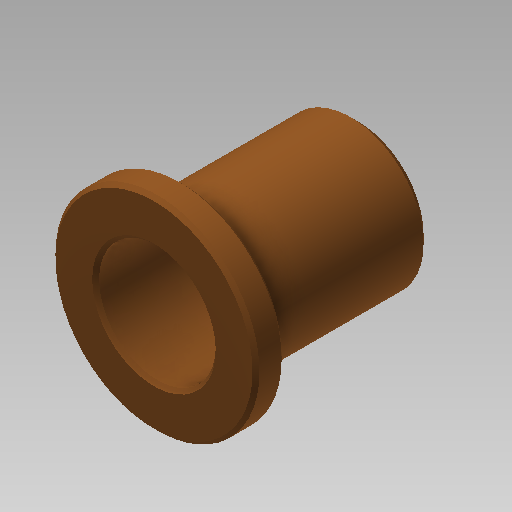
# Autodesk Inventor part: PWTR-0026
Saved by Autodesk Inventor 2020 (Build 240168000, 168)
## iProperties
Part Number: PWTR-0026
Document SubType Name: Modeling
Created: 2003-12-08
Designer: Bill Bogan
Material: Bronze, Soft Tin
Manufacturer: Standard
Standards Organization: Custom
Description: BUSHING - 1/2 ID
Density: 8.874 g/cm^3
Mass: 19.131 g
Surface Area: 25.0806 cm^2
Volume: 2.15584 cm^3
Appearance: Bronze - Satin
Vendor: Non-Design Specific
Control State: 0
Master: False
Checked Out: False
Shininess: 64.0
Length Units: 11272
Angle Units: 11279
Time Units: 11290
Mass Units: 11286
Length Display Precision: 3
Angle Display Precision: 2
Compacted: True
Today: Wednesday
Density: 0.0
Volumn: 0.0
Area: 0.0
PropertySet Name: Model Information
Author: Bill Bogan
Revision Number: B
Autodesk Inventor part; units mm, degrees
ref_plane "YZ Plane" through (0, 0, 0) normal (1, 0, 0) x (0, 1, 0)
ref_plane "XZ Plane" through (0, 0, 0) normal (0, 1, 0) x (-1, 0, 0)
ref_plane "XY Plane" through (0, 0, 0) normal (0, 0, 1) x (1, 0, 0)
sketch "Sketch1" plane through (0, 0, 0) normal (0, 0, 1) x (1, 0, 0)
  circle A0 centre (0, 0) radius 7.9375
  dimension "d0" = 15.875
  constraints: 1 centre point
  measures "d0" diameter of A0
extrude "Extrusion1" add sketch "Sketch1" along normal blind 19.05
sketch "Sketch2" plane through (0, 0, 19.05) normal (0, 0, 1) x (1, 0, 0)
  circle A0 centre (0, 0) radius 7.9375 projected
  circle A1 centre (0, 0) radius 11.1125
  dimension "d3" = 3.175
  constraints: 1 centre point
  measures "d3" radial gap between concentric circles of A0 A1
extrude "Extrusion2" add sketch "Sketch2" along normal blind 3.175 contours A0 | A1
chamfer "Chamfer1" distance 0.7937 angle 45 1 edges at (-7.9375, 0, 0)
sketch "Sketch3" plane through (0, 0, 22.225) normal (0, 0, 1) x (1, 0, 0)
  circle A0 centre (0, 0) radius 11.1125 projected
hole "Hole1" at (0, 0, 22.225) direction (0, 0, -1) diameter 12.7 end through all
chamfer "Chamfer2" distance 0.381 angle 45 2 edges at (0, 6.35, 22.225) (0, 6.35, 0)
chamfer "Chamfer3" distance 0.381 angle 45 2 edges at (-11.1125, 0, 22.225) (-11.1125, 0, 19.05)
body "Solid1"
